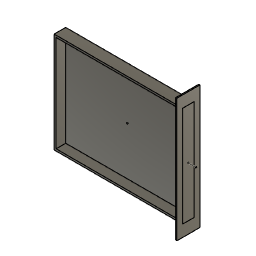
Behälter v2 (Autodesk Fusion 360 design; units mm, degrees)
Autodesk Fusion 360 part; units mm, degrees
sketch "Skizze1" plane through (0, 0, 0) normal (0, 1, 0) x (1, 0, 0)
  line L0 (-231.8939, 0) -> (98.1061, 0)
  line L1 (98.1061, 0) -> (98.1061, -260)
  line L2 (98.1061, -260) -> (-231.8939, -260)
  line L3 (-231.8939, -260) -> (-231.8939, 0)
  dimension "d1" = 260
  dimension "d2" = 330
  constraint horizontal L0
  constraint vertical L1
  constraint horizontal L2
  constraint vertical L3
  measures "d1" distance of L0.start L2.end
  measures "d2" distance of L1.end L2.end
extrude "Extrusion1" add sketch "Skizze1" along normal blind 30 makes body 1
shell "Schale1" thickness 5 removed faces 1 at (-121.8939, 0, 173.3333) on bodies 1
sketch "Skizze2" plane through (0, 30, 0) normal (0, 1, 0) x (-1, 0, 0)
  line L0 (231.8939, 260) -> (-98.1061, 260)
  line L1 (-98.1061, 260) -> (-98.1061, 0)
  line L2 (-98.1061, 0) -> (231.8939, 0)
  line L3 (231.8939, 0) -> (231.8939, 260)
  circle A0 centre (66.8939, 130) radius 3.5
  dimension "d6" = 7
  dimension "d7" = 130
  dimension "d8" = 130
  dimension "d9" = 165
  dimension "d10" = 165
  measures "d6" diameter of A0
  measures "d7" distance of L0 A0.centre
  measures "d8" distance of L2 A0.centre
  measures "d9" distance of L1 A0.centre
  measures "d10" distance of L3 A0.centre
extrude "Extrusion2" add sketch "Skizze2" along normal blind 15 contours A0 bodies 1
hole "Bohrung1" at (-66.8939, 45, 130) direction (0, -1, 0) diameter 4 depth 100 tip angle 180 bodies 1
sketch "Skizze3" plane through (98.1061, 0, 0) normal (1, 0, 0) x (0, 1, 0)
  line L0 (0, 260) -> (0, 0)
  line L1 (0, 0) -> (30, 0)
  line L2 (30, 0) -> (30, 260)
  line L3 (30, 260) -> (0, 260)
  line L4 (-15, 290) -> (45, 290)
  line L5 (45, 290) -> (45, -30)
  line L6 (45, -30) -> (-15, -30)
  line L7 (-15, -30) -> (-15, 290)
  dimension "d16" = 30
  dimension "d17" = 30
  dimension "d18" = 15
  dimension "d19" = 15
  constraint horizontal L4
  constraint vertical L5
  constraint horizontal L6
  constraint vertical L7
  measures "d16" distance of L3 L4
  measures "d17" distance of L1 L6
  measures "d18" distance of L0 L7
  measures "d19" distance of L2 L5
extrude "Extrusion3" add sketch "Skizze3" along normal blind 3 separate body makes body 2
move_face "Flächen versetzen1" offset 3 1 faces at (98.1061, 10, 86.6667) on bodies 1
sketch "Skizze4" plane through (101.1061, 0, 0) normal (1, 0, 0) x (0, 1, 0)
  line L0 (0, 260) -> (0, 0)
  line L1 (0, 0) -> (30, 0)
  line L2 (30, 0) -> (30, 260)
  line L3 (30, 260) -> (0, 260)
  circle A0 centre (15, 130) radius 1.5
  dimension "d23" = 3
  dimension "d24" = 130
  dimension "d25" = 130
  dimension "d26" = 15
  dimension "d27" = 15
  measures "d23" diameter of A0
  measures "d24" distance of L3 A0.centre
  measures "d25" distance of L1 A0.centre
  measures "d26" distance of L0 A0.centre
  measures "d27" distance of L2 A0.centre
extrude "Extrusion4" add sketch "Skizze4" along normal blind 20 contours A0 bodies 1
